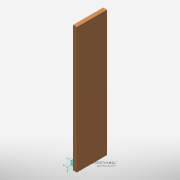
# Autodesk Inventor part: MPX-rib3
Saved by Autodesk Inventor 2016 (Build 200138000, 138)
## iProperties
Created: 2015-05-27
Part Number: MPX-rib3
Material: Wood (Cherry)
Document SubType Name: Modeling
Designer: as
Mass: 567 g
Surface Area: 1386 cm^2
Volume: 900 cm^3
Density: 0.63 g/cm^3
Appearance: Cherry - Natural Low Gloss
Author: as
Autodesk Inventor part; units mm, degrees
ref_plane "YZ Plane" through (0, 0, 0) normal (1, 0, 0) x (0, 1, 0)
ref_plane "XZ Plane" through (0, 0, 0) normal (0, 1, 0) x (-1, 0, 0)
ref_plane "XY Plane" through (0, 0, 0) normal (0, 0, 1) x (1, 0, 0)
sketch "Sketch1" plane through (0, 0, 0) normal (0, 0, 1) x (1, 0, 0)
  line L0 (0, 0) -> (-15, 0)
  line L1 (-15, 0) -> (-15, 120)
  line L2 (-15, 120) -> (0, 120)
  line L3 (0, 120) -> (0, 0)
  dimension "d0" = 15
  dimension "d1" = 120
  constraints: 8 end point, 2 parallel, 1 horizontal, 1 perpendicular
  measures "d0" distance of L1.end L2.end
  measures "d1" distance of L0.end L1.end
extrude "Extrusion1" add sketch "Sketch1" along normal blind 500
ref_plane "Work Plane1" through (0, 0, 250) normal (0, 0, -1) x (-1, 0, 0)
body "Solid1"
